Autodesk Inventor part; units mm, degrees
(part 2 of 2)
sketch "Sketch27" plane through (0, 0, 82.55) normal (0, 0, 1) x (1, 0, 0)
  line L0 (28.0831, 28.3843) -> (-28.0831, 28.3843) projected
  line L1 (25.1621, 23.6218) -> (25.1621, 26.9238) projected
  line L2 (14.5254, 18.8593) -> (-23.5746, 18.8593)
  line L3 (-23.5746, 18.8593) -> (-23.5746, 28.3843)
  line L4 (28.0831, 28.3843) -> (-28.0831, 28.3843) projected
  line L5 (-25.1621, 28.3843) -> (-25.1621, 17.2718)
  line L6 (-25.1621, 17.2718) -> (16.1129, 17.2718)
  line L7 (-25.1621, 28.3843) -> (-23.5746, 28.3843)
  line L8 (26.7496, 28.3843) -> (25.1621, 28.3843)
  line L9 (14.5254, 28.3843) -> (14.5254, 18.8593)
  line L10 (16.1129, 17.2718) -> (16.1129, 28.3843)
  line L11 (16.1129, 28.3843) -> (14.5254, 28.3843)
  point P0 (0, 0)
  point P1 (-25.1621, 26.9238)
  dimension "d85" = 1.5875
  dimension "d86" = 1.5875
  dimension "d88" = 9.525
  dimension "d96" = 38.1
  dimension "d97" = 1.5875
  constraints: 18 end point, 5 point on line, 3 collinear, 3 perpendicular, 2 vertical alignment, 1 vertical
  measures "d85" distance between parallel lines of L6 L2
  measures "d86" distance between parallel lines of L5 L3
  measures "d88" distance between parallel lines of L2 L0
  measures "d96" distance of L9.start L3.end
  measures "d97" distance of L10.end L9.start
extrude "Extrusion23" add sketch "Sketch27" against normal blind 66.675 contours L10 L6 L5 L0 L3 L2 L9
sketch "Sketch28" plane through (0, 0, 82.55) normal (0, 0, 1) x (1, 0, 0)
  circle A0 centre (-28.0831, 23.6218) radius 1.5875 projected
  arc A1 (29.6706, 23.6218) -> (29.6706, 23.6218) centre (28.0831, 23.6218) ccw projected
  circle A2 centre (28.0831, -23.6218) radius 1.5875 projected
  circle A3 centre (-28.0831, -23.6218) radius 1.5875 projected
  circle A4 centre (-28.0831, 23.6218) radius 1.27
  arc A5 (29.6706, 23.6218) -> (29.6706, 23.6218) centre (28.0831, 23.6218) ccw projected
  circle A6 centre (28.0831, 23.6218) radius 1.27
  circle A7 centre (28.0831, -23.6218) radius 1.5875 projected
  circle A8 centre (28.0831, -23.6218) radius 1.27
  circle A9 centre (-28.0831, -23.6218) radius 1.5875 projected
  circle A10 centre (-28.0831, -23.6218) radius 1.27
  line L0 (29.6706, 23.6218) -> (29.6706, 23.6218)
  line L1 (-23.5746, 26.9238) -> (14.5254, 26.9238) projected
  line L2 (14.5254, 26.9238) -> (14.5254, 18.8593) projected
  line L3 (14.5254, 18.8593) -> (-23.5746, 18.8593) projected
  line L4 (-23.5746, 18.8593) -> (-23.5746, 26.9238) projected
  line L5 (-25.1621, 23.6218) -> (-25.1621, 17.2718) projected
  line L6 (-25.1621, 17.2718) -> (16.1129, 17.2718) projected
  line L7 (16.1129, 17.2718) -> (16.1129, 26.9238) projected
  line L8 (16.1129, 26.9238) -> (25.1621, 26.9238) projected
  line L9 (25.1621, 26.9238) -> (25.1621, 23.6218) projected
  arc A11 (25.1621, 23.6218) -> (28.0831, 20.7008) centre (28.0831, 23.6218) ccw projected
  line L10 (28.0831, 20.7008) -> (31.3851, 20.7008) projected
  line L11 (31.3851, 20.7008) -> (31.3851, -20.7008) projected
  line L12 (31.3851, -20.7008) -> (28.0831, -20.7008) projected
  arc A12 (28.0831, -20.7008) -> (25.1621, -23.6218) centre (28.0831, -23.6218) ccw projected
  line L13 (25.1621, -23.6218) -> (25.1621, -26.9238) projected
  line L14 (25.1621, -26.9238) -> (10.795, -26.9238) projected
  line L15 (10.795, -26.9238) -> (10.795, -28.3843) projected
  line L16 (10.795, -28.3843) -> (-10.795, -28.3843) projected
  line L17 (-10.795, -28.3843) -> (-10.795, -26.9238) projected
  line L18 (-10.795, -26.9238) -> (-25.1621, -26.9238) projected
  line L19 (-25.1621, -26.9238) -> (-25.1621, -23.6218) projected
  arc A13 (-25.1621, -23.6218) -> (-28.0831, -20.7008) centre (-28.0831, -23.6218) ccw projected
  line L20 (-28.0831, -20.7008) -> (-31.3851, -20.7008) projected
  line L21 (-31.3851, -20.7008) -> (-31.3851, 20.7008) projected
  line L22 (-31.3851, 20.7008) -> (-28.0831, 20.7008) projected
  arc A14 (-28.0831, 20.7008) -> (-25.1621, 23.6218) centre (-28.0831, 23.6218) ccw projected
  line L23 (28.0831, 29.9718) -> (-28.0831, 29.9718) projected
  arc A15 (-28.0831, 29.9718) -> (-34.4331, 23.6218) centre (-28.0831, 23.6218) ccw projected
  line L24 (-34.4331, 23.6218) -> (-34.4331, -23.6218) projected
  arc A16 (-34.4331, -23.6218) -> (-28.0831, -29.9718) centre (-28.0831, -23.6218) ccw projected
  line L25 (-28.0831, -29.9718) -> (28.0831, -29.9718) projected
  arc A17 (28.0831, -29.9718) -> (34.4331, -23.6218) centre (28.0831, -23.6218) ccw projected
  line L26 (34.4331, -23.6218) -> (34.4331, 23.6218) projected
  arc A18 (34.4331, 23.6218) -> (28.0831, 29.9718) centre (28.0831, 23.6218) ccw projected
  circle A19 centre (28.0831, -23.6218) radius 1.5875 projected
  circle A20 centre (28.0831, 23.6218) radius 1.5875 projected
  circle A21 centre (-28.0831, 23.6218) radius 1.5875 projected
  circle A22 centre (-28.0831, -23.6218) radius 1.5875 projected
  point P0 (0, 0)
  dimension "d91" = 2.54
  constraints: 4 centre point, 4 coincident, 3 equal radius, 2 end point, 1 vertical
  measures "d91" diameter of A4
extrude "Extrusion24" add sketch "Sketch28" against normal blind 6.35 contours A0 | A1 | A2 | A3
sketch "Sketch29" plane through (0, 0, 76.2) normal (0, 0, -1) x (-1, 0, 0)
  line L0 (23.5746, 26.9238) -> (23.5746, 28.3843) projected
  line L1 (25.1621, 28.3843) -> (28.0831, 28.3843) projected
  line L2 (-25.1621, 23.6218) -> (-25.1621, 26.9238) projected
  line L3 (-14.5254, 26.9238) -> (23.5746, 26.9238) projected
  line L4 (-16.1129, 26.9238) -> (-16.1129, 28.3843) projected
  line L5 (-28.0831, 28.3843) -> (-16.1129, 28.3843) projected
  arc A0 (-28.0831, 28.3843) -> (-32.8456, 23.6218) centre (-28.0831, 23.6218) ccw projected
  line L6 (-32.8456, -23.6218) -> (-32.8456, 23.6218) projected
  arc A1 (-32.8456, -23.6218) -> (-28.0831, -28.3843) centre (-28.0831, -23.6218) ccw projected
  line L7 (-10.795, -28.3843) -> (-28.0831, -28.3843) projected
  line L8 (-10.795, -28.3843) -> (-10.795, -26.9238) projected
  line L9 (-10.795, -26.9238) -> (-25.1621, -26.9238) projected
  line L10 (-25.1621, -26.9238) -> (-25.1621, -23.6218) projected
  arc A2 (-25.1621, -23.6218) -> (-28.0831, -20.7008) centre (-28.0831, -23.6218) ccw projected
  line L11 (-28.0831, -20.7008) -> (-31.3851, -20.7008) projected
  line L12 (-31.3851, -20.7008) -> (-31.3851, 20.7008) projected
  line L13 (-31.3851, 20.7008) -> (-28.0831, 20.7008) projected
  arc A3 (-28.0831, 20.7008) -> (-25.1621, 23.6218) centre (-28.0831, 23.6218) ccw projected
  line L14 (-25.1621, 26.9238) -> (-16.1129, 26.9238) projected
  line L15 (25.1621, 28.3843) -> (25.1621, 23.6218) projected
  arc A4 (25.1621, 23.6218) -> (28.0831, 20.7008) centre (28.0831, 23.6218) ccw projected
  line L16 (28.0831, 20.7008) -> (31.3851, 20.7008) projected
  line L17 (31.3851, 20.7008) -> (31.3851, -20.7008) projected
  line L18 (31.3851, -20.7008) -> (28.0831, -20.7008) projected
  arc A5 (28.0831, -20.7008) -> (25.1621, -23.6218) centre (28.0831, -23.6218) ccw projected
  line L19 (25.1621, -23.6218) -> (25.1621, -26.9238) projected
  line L20 (25.1621, -26.9238) -> (10.795, -26.9238) projected
  line L21 (10.795, -26.9238) -> (10.795, -28.3843) projected
  line L22 (28.0831, -28.3843) -> (10.795, -28.3843) projected
  arc A6 (28.0831, -28.3843) -> (32.8456, -23.6218) centre (28.0831, -23.6218) ccw projected
  line L23 (32.8456, 23.6218) -> (32.8456, -23.6218) projected
  arc A7 (32.8456, 23.6218) -> (28.0831, 28.3843) centre (28.0831, 23.6218) ccw projected
  line L24 (-14.5254, 28.3843) -> (23.5746, 28.3843) projected
  line L25 (-14.5254, 28.3843) -> (-14.5254, 26.9238) projected
  point P0 (0, 0)
extrude "Extrusion25" cut sketch "Sketch29" against normal blind 6.35 contours L3 L25 L24 L0
sketch "Sketch30" plane through (0, 0, 82.55) normal (0, 0, 1) x (1, 0, 0)
  arc A0 (30.1353, -1.8899) -> (23.4472, 16.9713) centre (20.8658, 5.4396) ccw projected
  arc A1 (30.2628, -1.9908) -> (23.4827, 17.13) centre (20.8658, 5.4396) ccw
  line L0 (32.8456, -23.6218) -> (32.8456, 23.6218) projected
  line L1 (30.2628, -1.9908) -> (23.4827, 17.13)
  point P0 (0, 0)
  constraints: 2 end point, 2 point on circle, 1 centre point, 1 tangent
extrude "Extrusion26" cut sketch "Sketch30" against normal blind 6.35
sketch "Sketch31" plane through (-12.9718, -22.0343, 11.1882) normal (0, 1, 0) x (1, 0, 0)
  line L0 (29.845, 0) -> (29.845, 6.35) projected
  line L1 (-1.905, 6.35) -> (-1.905, 0) projected
  line L2 (11.43, -0.4687) -> (16.51, -0.4687) projected
  line L3 (7.62, 6.35) -> (5.08, 6.35) projected
  line L4 (-1.905, 0) -> (7.62, 0)
  line L5 (7.62, 0) -> (7.62, 6.35)
  line L6 (7.62, 6.35) -> (-1.905, 6.35)
  line L7 (-1.905, 6.35) -> (-1.905, 0)
  line L8 (31.75, 0) -> (-3.81, 0) projected
  line L9 (29.845, 6.35) -> (20.32, 6.35)
  line L10 (20.32, 6.35) -> (20.32, 0)
  line L11 (20.32, 0) -> (29.845, 0)
  line L12 (29.845, 0) -> (29.845, 6.35)
  point P0 (12.9718, 11.1882)
  constraints: 16 end point, 4 parallel, 2 horizontal, 2 perpendicular, 1 collinear, 1 point on line
extrude "Extrusion27" add sketch "Sketch31" along normal up to surface (50.4186 mm away)
sketch "Sketch32" plane through (-12.9718, -22.0343, 11.1882) normal (0, -1, 0) x (1, 0, 0)
  line L0 (27.94, -6.35) -> (27.94, 0) projected
  line L1 (29.845, -6.35) -> (27.94, -6.35) projected
  line L2 (29.845, 0) -> (29.845, -6.35) projected
  line L3 (27.94, 0) -> (29.845, 0) projected
  line L4 (0, 0) -> (0, -6.35) projected
  line L5 (-1.905, 0) -> (0, 0) projected
  line L6 (-1.905, -6.35) -> (-1.905, 0) projected
  line L7 (0, -6.35) -> (-1.905, -6.35) projected
  point P0 (12.9718, -11.1882)
extrude "Extrusion28" add sketch "Sketch32" along normal blind 2.54
sketch "Sketch33" plane through (-14.8768, -28.3843, 4.8382) normal (0, 0, -1) x (-1, 0, 0)
  circle A0 centre (-11.3674, 18.48) radius 1.5875 projected
  circle A1 centre (-15.875, 13.97) radius 2.54 projected
  circle A2 centre (-28.575, 24.765) radius 1.397 projected
  circle A3 centre (-3.175, 24.765) radius 1.397 projected
  circle A4 centre (-15.875, 20.955) radius 2.286 projected
  circle A5 centre (-3.175, 3.175) radius 1.397 projected
  circle A6 centre (-28.575, 3.175) radius 1.397 projected
  line L0 (-28.575, 12.7) -> (-28.575, 15.24) projected
  line L1 (-28.575, 12.7) -> (-31.3246, 7.9375) projected
  arc A7 (-31.3246, 7.9375) -> (-31.75, 6.35) centre (-28.575, 6.35) ccw projected
  line L2 (-31.75, 6.35) -> (-31.75, 0) projected
  line L3 (-31.75, 0) -> (0, 0) projected
  line L4 (0, 0) -> (0, 6.35) projected
  arc A8 (0, 6.35) -> (-0.4254, 7.9375) centre (-3.175, 6.35) ccw projected
  line L5 (-0.4254, 7.9375) -> (-3.175, 12.7) projected
  line L6 (-3.175, 12.7) -> (-3.175, 15.24) projected
  line L7 (-0.4254, 20.0025) -> (-3.175, 15.24) projected
  arc A9 (-0.4254, 20.0025) -> (0, 21.59) centre (-3.175, 21.59) ccw projected
  line L8 (0, 27.94) -> (0, 21.59) projected
  line L9 (-31.75, 27.94) -> (0, 27.94) projected
  line L10 (-31.75, 21.59) -> (-31.75, 27.94) projected
  arc A10 (-31.75, 21.59) -> (-31.3246, 20.0025) centre (-28.575, 21.59) ccw projected
  line L11 (-28.575, 15.24) -> (-31.3246, 20.0025) projected
  circle A11 centre (-15.875, 6.985) radius 2.286 projected
  circle A12 centre (-3.175, 3.175) radius 1.27
  circle A13 centre (-28.575, 3.175) radius 1.27
  circle A14 centre (-28.575, 24.765) radius 1.27
  circle A15 centre (-3.175, 24.765) radius 1.27
  point P0 (-14.8768, 28.3843)
  dimension "d104" = 2.54
  constraints: 4 centre point, 4 coincident, 3 equal radius
  measures "d104" diameter of A12
extrude "Extrusion29" cut sketch "Sketch33" against normal through all contours A12 | A13 | A14 | A15
sketch "Sketch34" plane through (0, 0, 15.875) normal (0, 0, -1) x (-1, 0, 0)
  line L0 (-16.1129, 28.3843) -> (-14.5254, 28.3843) projected
  line L1 (-16.1129, 28.3843) -> (-16.1129, 17.2718) projected
  line L2 (-16.1129, 17.2718) -> (25.1621, 17.2718) projected
  line L3 (25.1621, 17.2718) -> (25.1621, 28.3843) projected
  line L4 (23.5746, 28.3843) -> (25.1621, 28.3843) projected
  line L5 (23.5746, 28.3843) -> (23.5746, 18.8593) projected
  line L6 (23.5746, 18.8593) -> (-14.5254, 18.8593) projected
  line L7 (-14.5254, 18.8593) -> (-14.5254, 28.3843) projected
  point P0 (0, 0)
extrude "Extrusion30" add sketch "Sketch34" along normal up to surface (4.6868 mm away)
sketch "Sketch35" plane through (-14.8768, -28.3843, 4.8382) normal (0, 0, -1) x (-1, 0, 0)
  line L0 (-9.525, 6.35) -> (-9.525, 56.7686) projected
  line L1 (-9.525, 31.5593) -> (-22.225, 31.5593)
  line L2 (-22.225, 31.5593) -> (-22.225, 56.8713)
  line L3 (-22.225, 56.8713) -> (-9.525, 56.8713)
  line L4 (-9.525, 56.8713) -> (-9.525, 31.5593)
  line L5 (-22.225, 6.35) -> (-22.225, 56.7686) projected
  point P0 (-14.8768, 28.3843)
  point P1 (-22.225, 31.5593)
  constraints: 8 end point, 2 midpoint, 2 parallel, 1 coincident, 1 horizontal, 1 perpendicular
extrude "Extrusion31" add sketch "Sketch35" against normal up to surface (6.35 mm away)
sketch "Sketch36" plane through (-14.8768, -28.3843, 4.8382) normal (0, 0, -1) x (-1, 0, 0)
  arc A0 (13.2062, -1.5875) -> (19.5562, 4.7625) centre (13.2062, 4.7625) ccw projected
  line L0 (19.5562, 52.0061) -> (19.5562, 4.7625) projected
  arc A1 (19.5562, 52.0061) -> (13.2062, 58.3561) centre (13.2062, 52.0061) ccw projected
  line L1 (-42.9599, 58.3561) -> (13.2062, 58.3561) projected
  arc A2 (-42.9599, 58.3561) -> (-49.3099, 52.0061) centre (-42.9599, 52.0061) ccw projected
  line L2 (-49.3099, 4.7625) -> (-49.3099, 52.0061) projected
  arc A3 (-49.3099, 4.7625) -> (-42.9599, -1.5875) centre (-42.9599, 4.7625) ccw projected
  line L3 (13.2062, -1.5875) -> (-42.9599, -1.5875) projected
  circle A4 centre (-42.9599, 4.7625) radius 1.5875 projected
  circle A5 centre (-42.9599, 52.0061) radius 1.5875 projected
  circle A6 centre (13.2062, 52.0061) radius 1.5875 projected
  line L4 (-40.0389, 1.4605) -> (10.2852, 1.4605) projected
  line L5 (-40.0389, 1.4605) -> (-40.0389, 4.7625) projected
  arc A7 (-40.0389, 4.7625) -> (-42.9599, 7.6835) centre (-42.9599, 4.7625) ccw projected
  line L6 (-42.9599, 7.6835) -> (-46.2619, 7.6835) projected
  line L7 (-46.2619, 49.0851) -> (-46.2619, 7.6835) projected
  line L8 (-46.2619, 49.0851) -> (-42.9599, 49.0851) projected
  arc A8 (-42.9599, 49.0851) -> (-40.0389, 52.0061) centre (-42.9599, 52.0061) ccw projected
  line L9 (-40.0389, 52.0061) -> (-40.0389, 55.3081) projected
  line L10 (10.2852, 55.3081) -> (-40.0389, 55.3081) projected
  line L11 (10.2852, 55.3081) -> (10.2852, 52.0061) projected
  arc A9 (10.2852, 52.0061) -> (13.2062, 49.0851) centre (13.2062, 52.0061) ccw projected
  line L12 (13.2062, 49.0851) -> (16.5082, 49.0851) projected
  line L13 (16.5082, 7.6835) -> (16.5082, 49.0851) projected
  line L14 (16.5082, 7.6835) -> (13.2062, 7.6835) projected
  arc A10 (13.2062, 7.6835) -> (10.2852, 4.7625) centre (13.2062, 4.7625) ccw projected
  line L15 (10.2852, 4.7625) -> (10.2852, 1.4605) projected
  circle A11 centre (13.2062, 4.7625) radius 1.5875 projected
  line L16 (0, 56.7686) -> (0, 47.2436) projected
  line L17 (-42.9599, 58.3561) -> (13.2062, 58.3561) projected
  line L18 (0, 55.3081) -> (-31.75, 55.3081)
  line L19 (-31.75, 55.3081) -> (-31.75, 58.3561)
  line L20 (-31.75, 58.3561) -> (0, 58.3561)
  line L21 (0, 58.3561) -> (0, 55.3081)
  line L22 (-31.75, 1.905) -> (-31.75, 56.7686) projected
  line L23 (-31.75, 1.4605) -> (0, 1.4605)
  line L24 (0, 1.4605) -> (0, -1.5875)
  line L25 (0, -1.5875) -> (-31.75, -1.5875)
  line L26 (-31.75, -1.5875) -> (-31.75, 1.4605)
  point P0 (-14.8768, 28.3843)
  point P1 (-31.75, 29.3368)
  constraints: 16 end point, 5 point on line, 4 parallel, 2 horizontal, 2 perpendicular, 1 midpoint, 1 vertical alignment
extrude "Extrusion32" add sketch "Sketch36" along normal up to surface (4.8382 mm away) contours L3 L26 L4 L24 | L21 L16 L10 L19 L1
sketch "Sketch37" plane through (-14.8768, 17.2718, 11.1882) normal (0, 0, -1) x (-1, 0, 0)
  line L0 (0, 9.6647) -> (0, 11.1125) projected
  line L1 (10.2852, 0) -> (0, 0)
  line L2 (0, 0) -> (0, 11.1125)
  line L3 (0, 11.1125) -> (10.2852, 11.1125)
  line L4 (10.2852, 11.1125) -> (10.2852, 0)
  line L5 (0, 0) -> (10.2852, 0) projected
  point P0 (-14.8768, -17.2718)
  constraints: 8 end point, 2 parallel, 1 horizontal, 1 perpendicular
extrude "Extrusion33" add sketch "Sketch37" along normal blind 2.54
sketch "Sketch38" plane through (16.1129, 17.2718, 82.55) normal (1, 0, 0) x (0, 0, -1)
  line L0 (68.8788, 2.2475) -> (59.3538, 2.2475)
  line L1 (59.3538, 2.2475) -> (59.3538, 11.1125)
  line L2 (59.3538, 11.1125) -> (68.8788, 11.1125)
  line L3 (68.8788, 11.1125) -> (68.8788, 2.2475)
  line L4 (6.35, 11.1125) -> (71.3618, 11.1125) projected
  point P0 (82.55, -17.2718)
  dimension "d115" = 9.525
  constraints: 8 end point, 2 parallel, 1 collinear, 1 horizontal, 1 perpendicular
  measures "d115" distance of L0.start L0.end
extrude "Extrusion34" cut sketch "Sketch38" against normal blind 2.54
chamfer "Chamfer3" distance 3.175 angle 45 1 edges at (-14.8768, 22.8281, 8.6482)
sketch "Sketch39" plane through (-14.8768, -28.3843, 4.8382) normal (0, 0, -1) x (-1, 0, 0)
  line L0 (-9.525, 31.5593) -> (-22.225, 31.5593) projected
  line L1 (-22.225, 31.5593) -> (-9.525, 31.5593)
  line L2 (-9.525, 31.5593) -> (-9.525, 37.929)
  line L3 (-9.525, 37.929) -> (-22.225, 37.929)
  line L4 (-22.225, 37.929) -> (-22.225, 31.5593)
  point P0 (-14.8768, 28.3843)
  constraints: 8 end point, 2 parallel, 1 horizontal, 1 perpendicular
extrude "Extrusion35" cut sketch "Sketch39" against normal through all
sketch "Sketch40" plane through (-14.8768, -28.3843, 4.8382) normal (0, 0, -1) x (-1, 0, 0)
  line L0 (5.27, 28.402) -> (-12.1771, 28.402)
  line L1 (-12.1771, 28.402) -> (-12.1771, 43.2086)
  line L2 (-12.1771, 43.2086) -> (5.27, 43.2086)
  line L3 (5.27, 43.2086) -> (5.27, 28.402)
  point P0 (-14.8768, 28.3843)
  constraints: 8 end point, 2 parallel, 1 horizontal, 1 perpendicular
extrude "Extrusion36" [suppressed]
sketch "Sketch41" plane through (0, 0, 0) normal (0, 0, -1) x (-1, 0, 0)
  line L0 (-25.1595, -3.0552) -> (25.1489, -3.0552)
  line L1 (25.1489, -3.0552) -> (25.1489, -28.4414)
  line L2 (25.1489, -28.4414) -> (-25.1595, -28.4414)
  line L3 (-25.1595, -28.4414) -> (-25.1595, -3.0552)
  point P0 (0, 0)
  constraints: 8 end point, 2 parallel, 1 horizontal, 1 perpendicular
extrude "Extrusion37" cut sketch "Sketch41" against normal up to surface (4.8382 mm away)
body "Solid1"
